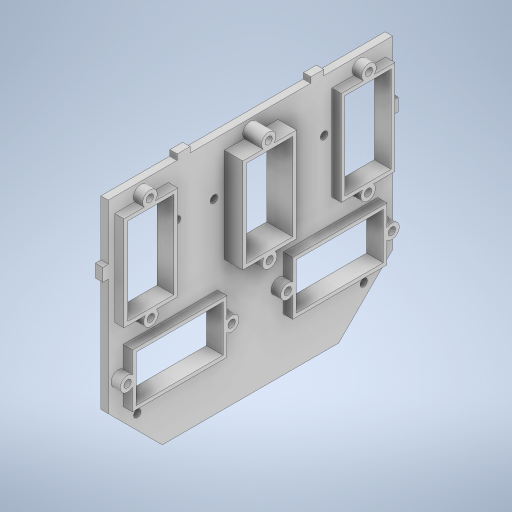
# Autodesk Inventor part: Palm_ServoAttachment
Saved by Autodesk Inventor 2023 (Build 270158000, 158)
## iProperties
Created: 2023-04-20
Part Number: Palm_ServoAttachment
Material: Generic
Document SubType Name: Modeling
Designer: 1senadi
Density: 1 g/cm^3
Appearance: Default
Author: 1senadi
Autodesk Inventor part; units mm, degrees
ref_plane "YZ Plane" through (0, 0, 0) normal (1, 0, 0) x (0, 1, 0)
ref_plane "XZ Plane" through (0, 0, 0) normal (0, 1, 0) x (-1, 0, 0)
ref_plane "XY Plane" through (0, 0, 0) normal (0, 0, 1) x (1, 0, 0)
sketch "Sketch1" plane through (0, 0, 0) normal (1, 0, 0) x (0, 1, 0)
  line L0 (0, 0) -> (0, -76.8)
  line L1 (0, 0) -> (76.8, 0) construction
  line L2 (0, -76.8) -> (-50, -76.8)
  line L3 (-50, -76.8) -> (-50, 0)
  line L4 (-50, 0) -> (0, 0)
  dimension "d0" = 76.8
  dimension "d1" = 90
  dimension "d2" = 50
  constraints: 10 end point, 3 perpendicular, 2 horizontal, 1 vertical
  measures "d0" distance of L0.start L0.end
  measures "d1" angle of L0 L1
  measures "d2" distance of L0.end L2.end
extrude "Extrusion1" add sketch "Sketch1" along normal blind 2
sketch "Sketch2" plane through (0, 0, 0) normal (-1, 0, 0) x (0, 0, 1)
  line L0 (-76.8, -50) -> (-76.8, 0) projected
  line L1 (-76.8, 0) -> (-73.92, 0)
  line L2 (-76.8, 0) -> (0, 0) projected
  line L3 (-73.92, 0) -> (-73.92, -5)
  line L4 (-73.92, -5) -> (-61.42, -5)
  line L5 (-61.42, -5) -> (-61.42, -28.5)
  line L6 (-61.42, -28.5) -> (-73.92, -28.5)
  line L7 (-73.92, -28.5) -> (-73.92, -5)
  line L8 (-73.92, -5) -> (-38.32, -5)
  line L9 (-38.32, -5) -> (-2.72, -5)
  line L10 (-2.72, -5) -> (-2.72, -28.5)
  line L11 (-2.72, -28.5) -> (-15.22, -28.5)
  line L12 (-15.22, -28.5) -> (-15.22, -5)
  line L13 (-38.32, -5) -> (-32.32, -5)
  line L14 (-32.32, -5) -> (-32.32, -28.5)
  line L15 (-32.32, -28.5) -> (-44.82, -28.5)
  line L16 (-44.82, -28.5) -> (-44.82, -5)
  line L17 (-67.67, -28.5) -> (-67.67, -30.813)
  line L18 (-67.92, -5) -> (-67.92, -2.687)
  circle A0 centre (-67.92, -2.687) radius 1
  circle A1 centre (-67.67, -30.813) radius 1
  line L19 (-38.57, -28.5) -> (-38.57, -30.813)
  line L20 (-38.32, -5) -> (-38.32, -2.687)
  line L21 (-8.72, -5) -> (-8.72, -2.687)
  line L22 (-8.97, -28.5) -> (-8.97, -30.813)
  circle A2 centre (-38.32, -2.687) radius 1
  circle A3 centre (-8.72, -2.687) radius 1
  circle A4 centre (-38.57, -30.813) radius 1
  circle A5 centre (-8.97, -30.813) radius 1
  dimension "d5" = 2.88
  dimension "d6" = 5
  dimension "d7" = 12.5
  dimension "d8" = 23.5
  dimension "d9" = 12.5
  dimension "d10" = 35.6
  dimension "d14" = 35.6
  dimension "d15" = 23.5
  dimension "d16" = 12.5
  dimension "d17" = 6
  dimension "d18" = 23.5
  dimension "d19" = 12.5
  dimension "d24" = 2.313
  dimension "d25" = 2.313
  dimension "d26" = 2
  dimension "d27" = 2
  dimension "d28" = 2
  dimension "d29" = 2
  dimension "d30" = 2
  dimension "d31" = 2
  constraints: 42 end point, 9 perpendicular, 6 centre point, 6 coincident, 6 point on line, 6 vertical, 3 horizontal, 3 midpoint
  measures "d5" distance of L0.end L1.end
  measures "d6" distance of L1.end L3.end
  measures "d7" distance of L3.end L4.end
  measures "d8" distance of L4.end L5.end
  measures "d9" distance of L5.end L6.end
  measures "d10" distance of L3.end L8.end
  measures "d14" distance of L8.end L9.end
  measures "d15" distance of L9.end L10.end
  measures "d16" distance of L10.end L11.end
  measures "d17" distance of L8.end L13.end
  measures "d18" distance of L13.end L14.end
  measures "d19" distance of L14.end L15.end
  measures "d24" distance of L17.start L17.end
  measures "d25" distance of L18.start L18.end
  measures "d26" diameter of A0
  measures "d27" diameter of A1
  measures "d28" diameter of A2
  measures "d29" diameter of A3
  measures "d30" diameter of A4
  measures "d31" diameter of A5
extrude "Extrusion2" cut sketch "Sketch2" against normal up to surface (2 mm away)
sketch "Sketch8" plane through (2, 0, 0) normal (1, 0, 0) x (0, 0, -1)
  line L0 (0, 0) -> (0, -50) projected
  line L1 (0, 0) -> (0, -15)
  line L2 (0, -15) -> (0, -18.5)
  line L3 (0, -18.5) -> (-1.5, -18.5)
  line L4 (-1.5, -18.5) -> (-1.5, -15)
  line L5 (-1.5, -15) -> (0, -15)
  line L6 (0, 0) -> (18.6, 0)
  line L7 (76.8, 0) -> (0, 0) projected
  line L8 (18.6, 0) -> (22.1, 0)
  line L9 (22.1, 0) -> (22.1, 1.5)
  line L10 (22.1, 1.5) -> (18.6, 1.5)
  line L11 (18.6, 1.5) -> (18.6, 0)
  line L12 (0, -50) -> (76.8, -50) projected
  line L13 (38.4, -50) -> (38.4, 0)
  line L14 (76.8, -15) -> (76.8, -18.5)
  line L15 (76.8, -18.5) -> (78.3, -18.5)
  line L16 (78.3, -18.5) -> (78.3, -15)
  line L17 (78.3, -15) -> (76.8, -15)
  line L18 (58.2, 0) -> (54.7, 0)
  line L19 (54.7, 0) -> (54.7, 1.5)
  line L20 (54.7, 1.5) -> (58.2, 1.5)
  line L21 (58.2, 1.5) -> (58.2, 0)
  dimension "d63" = 15
  dimension "d64" = 3.5
  dimension "d65" = 1.5
  dimension "d66" = 3.5
  dimension "d67" = 18.6
  dimension "d68" = 3.5
  dimension "d69" = 1.5
  dimension "d70" = 3.5
  constraints: 38 end point, 8 symmetric about line, 5 point on line, 4 perpendicular, 1 midpoint, 1 parallel
  measures "d63" distance of L0.start L1.end
  measures "d64" distance of L1.end L2.end
  measures "d65" distance of L2.end L3.end
  measures "d66" distance of L3.end L4.end
  measures "d67" distance of L0.start L6.end
  measures "d68" distance of L6.end L8.end
  measures "d69" distance of L8.end L9.end
  measures "d70" distance of L9.end L10.end
extrude "Extrusion7" add sketch "Sketch8" against normal up to surface (2 mm away) contours L0 L3 L4 L5 | L11 L10 L9 L7 | L7 L19 L20 L21 | L17 L16 L15 L14
sketch "Sketch10" plane through (2, 0, 0) normal (1, 0, 0) x (0, 0, -1)
  circle A0 centre (8.97, -30.813) radius 1 projected
  line L0 (0, -18.5) -> (0, -50) projected
  line L1 (8.72, -31.813) -> (0, -31.813)
  line L2 (0, -31.813) -> (0, -36.813)
  line L3 (0, -36.813) -> (5, -36.813)
  line L4 (5, -36.813) -> (5, -49.313)
  line L5 (5, -49.313) -> (28.5, -49.313)
  line L6 (5, -49.313) -> (28.5, -49.313) construction
  line L7 (28.5, -49.313) -> (28.5, -36.813)
  line L8 (28.5, -36.813) -> (5, -36.813)
  line L9 (5, -43.063) -> (2.687, -43.063)
  line L10 (28.5, -43.063) -> (30.813, -43.063)
  circle A1 centre (2.687, -43.063) radius 1
  circle A2 centre (30.813, -43.063) radius 1
  line L11 (54.7, 0) -> (22.1, 0) projected
  line L12 (38.4, 0) -> (38.4, -50)
  line L13 (71.8, -36.813) -> (71.8, -49.313)
  line L14 (71.8, -49.313) -> (48.3, -49.313)
  line L15 (48.3, -49.313) -> (48.3, -36.813)
  line L16 (48.3, -36.813) -> (71.8, -36.813)
  line L17 (71.8, -43.063) -> (74.113, -43.063)
  line L18 (48.3, -43.063) -> (45.987, -43.063)
  circle A3 centre (74.113, -43.063) radius 1
  circle A4 centre (45.987, -43.063) radius 1
  point P0 (0, 0)
  dimension "d82" = 5
  dimension "d83" = 5
  dimension "d84" = 12.5
  dimension "d85" = 23.5
  dimension "d86" = 0
  dimension "d87" = 12.5
  dimension "d88" = 2.313
  dimension "d89" = 2.313
  dimension "d90" = 2
  dimension "d91" = 2
  constraints: 34 end point, 10 symmetric about line, 4 centre point, 4 coincident, 4 horizontal, 3 midpoint, 3 perpendicular, 2 point on line, 2 vertical, 1 collinear, 2 other
  measures "d82" distance of L1.end L2.end
  measures "d83" distance of L2.end L3.end
  measures "d84" distance of L3.end L4.end
  measures "d85" distance of L4.end L5.end
  measures "d86" distance between parallel lines of L5 L6
  measures "d87" distance of L5.end L7.end
  measures "d88" distance of L9.start L9.end
  measures "d89" distance of L10.start L10.end
  measures "d90" diameter of A1
  measures "d91" diameter of A2
extrude "Extrusion8" cut sketch "Sketch10" against normal up to surface (2 mm away) contours L8 L7 L5 L4 | A1 | A2 | L13 L14 L15 L16 | A3 | A4
sketch "Sketch11" plane through (2, 0, 0) normal (1, 0, 0) x (0, 0, -1)
  line L0 (0, -50) -> (76.8, -50) projected
  line L1 (0, -50) -> (14.5664, -64.5664)
  line L2 (0, -50) -> (20.6, -50) construction
  line L3 (76.8, -50) -> (62.2336, -64.5664)
  line L4 (76.8, -50) -> (97.4, -50) construction
  line L5 (62.2336, -64.5664) -> (14.5664, -64.5664)
  point P0 (0, 0)
  dimension "d94" = 20.6
  dimension "d95" = 45
  dimension "d96" = 20.6
  dimension "d97" = 135
  constraints: 10 end point, 2 equal length, 2 horizontal
  measures "d94" distance of L0.start L1.end
  measures "d95" angle of L1 L2
  measures "d96" distance of L0.end L3.end
  measures "d97" angle of L3 L4
extrude "Extrusion9" add sketch "Sketch11" against normal up to surface (2 mm away)
sketch "Sketch12" plane through (2, 0, 0) normal (1, 0, 0) x (0, 0, -1)
  circle A0 centre (2.687, -43.063) radius 1 projected
  circle A1 centre (30.813, -43.063) radius 1 projected
  line L0 (5, -36.813) -> (28.5, -36.813) projected
  line L1 (5, -49.313) -> (5, -36.813) projected
  line L2 (28.5, -49.313) -> (5, -49.313) projected
  line L3 (28.5, -36.813) -> (28.5, -49.313) projected
  line L4 (29.5, -35.813) -> (4, -35.813)
  line L5 (4, -35.813) -> (4, -50.313)
  line L6 (4, -50.313) -> (29.5, -50.313)
  line L7 (29.5, -50.313) -> (29.5, -35.813)
  circle A2 centre (2.687, -43.063) radius 2
  circle A3 centre (30.813, -43.063) radius 2
  point P0 (0, 0)
  point P1 (4, -41.313)
  point P2 (4, -44.313)
  point P3 (29.5, -41.313)
  point P4 (29.5, -44.313)
  point P5 (4, -44.5717)
  point P6 (4, -41.5543)
  point P7 (29.5, -41.5543)
  point P8 (29.5, -44.5717)
  dimension "d102" = 1
  dimension "d110" = 1
  dimension "d111" = 1
  constraints: 8 end point, 4 point on line, 2 centre point, 3 other
  measures "d102" distance between parallel lines of L0 L4
  measures "d110" radial gap between concentric circles of A0 A2
  measures "d111" radial gap between concentric circles of A1 A3
extrude "Extrusion10" add sketch "Sketch12" along normal blind 2.5
sketch "Sketch13" plane through (2, 0, 0) normal (1, 0, 0) x (0, 0, -1)
  line L0 (48.3, -49.313) -> (48.3, -36.813) projected
  line L1 (48.3, -36.813) -> (71.8, -36.813) projected
  line L2 (71.8, -49.313) -> (48.3, -49.313) projected
  line L3 (71.8, -36.813) -> (71.8, -49.313) projected
  circle A0 centre (74.113, -43.063) radius 1 projected
  circle A1 centre (45.987, -43.063) radius 1 projected
  line L4 (47.3, -35.813) -> (47.3, -50.313)
  line L5 (47.3, -50.313) -> (72.8, -50.313)
  line L6 (72.8, -50.313) -> (72.8, -35.813)
  line L7 (72.8, -35.813) -> (47.3, -35.813)
  arc A2 (47.3, -41.5543) -> (47.3, -44.5717) centre (45.987, -43.063) ccw
  arc A3 (72.8, -44.5717) -> (72.8, -41.5543) centre (74.113, -43.063) ccw
  point P0 (0, 0)
  dimension "d105" = 1
  dimension "d106" = 1
  dimension "d107" = 1
  constraints: 8 end point, 4 point on circle, 4 point on line, 2 centre point, 3 other
  measures "d105" distance between parallel lines of L0 L4
  measures "d106" radial gap between concentric circles of A1 A2
  measures "d107" radial gap between concentric circles of A0 A3
extrude "Extrusion11" add sketch "Sketch13" along normal blind 2.5
sketch "Sketch14" plane through (2, 0, 0) normal (1, 0, 0) x (0, 0, -1)
  line L0 (2.72, -5) -> (15.22, -5) projected
  line L1 (2.72, -28.5) -> (2.72, -5) projected
  line L2 (15.22, -28.5) -> (2.72, -28.5) projected
  circle A0 centre (8.97, -30.813) radius 1 projected
  line L3 (15.22, -5) -> (15.22, -28.5) projected
  circle A1 centre (8.72, -2.687) radius 1 projected
  line L4 (16.22, -29.5) -> (1.72, -29.5)
  line L5 (1.72, -29.5) -> (1.72, -4)
  line L6 (1.72, -4) -> (16.22, -4)
  line L7 (16.22, -4) -> (16.22, -29.5)
  circle A2 centre (8.72, -2.687) radius 2
  circle A3 centre (8.97, -30.813) radius 2
  point P0 (0, 0)
  point P1 (10.2287, -4)
  point P2 (7.2113, -4)
  point P3 (7.4613, -29.5)
  point P4 (10.4787, -29.5)
  dimension "d112" = 1
  dimension "d113" = 1
  dimension "d114" = 1
  constraints: 8 end point, 2 centre point, 3 other
  measures "d112" distance between parallel lines of L3 L7
  measures "d113" radial gap between concentric circles of A1 A2
  measures "d114" radial gap between concentric circles of A0 A3
extrude "Extrusion12" add sketch "Sketch14" along normal blind 2.5
sketch "Sketch15" plane through (2, 0, 0) normal (1, 0, 0) x (0, 0, -1)
  line L0 (32.32, -5) -> (44.82, -5) projected
  line L1 (44.82, -5) -> (44.82, -28.5) projected
  line L2 (32.32, -28.5) -> (32.32, -5) projected
  line L3 (44.82, -28.5) -> (32.32, -28.5) projected
  circle A0 centre (38.57, -30.813) radius 1 projected
  circle A1 centre (38.32, -2.687) radius 1 projected
  line L4 (45.82, -29.5) -> (45.82, -4)
  line L5 (45.82, -4) -> (31.32, -4)
  line L6 (31.32, -4) -> (31.32, -29.5)
  line L7 (31.32, -29.5) -> (45.82, -29.5)
  circle A2 centre (38.32, -2.687) radius 2
  circle A3 centre (38.57, -30.813) radius 2
  point P0 (0, 0)
  point P1 (39.8287, -4)
  point P2 (36.8113, -4)
  point P3 (37.0613, -29.5)
  point P4 (40.0787, -29.5)
  dimension "d117" = 1
  dimension "d118" = 1
  dimension "d119" = 1
  constraints: 8 end point, 2 centre point, 3 other
  measures "d117" distance between parallel lines of L1 L4
  measures "d118" radial gap between concentric circles of A1 A2
  measures "d119" radial gap between concentric circles of A0 A3
extrude "Extrusion13" add sketch "Sketch15" along normal blind 5
sketch "Sketch16" plane through (2, 0, 0) normal (1, 0, 0) x (0, 0, -1)
  line L0 (61.42, -5) -> (73.92, -5) projected
  line L1 (73.92, -5) -> (73.92, -28.5) projected
  line L2 (61.42, -28.5) -> (61.42, -5) projected
  line L3 (73.92, -28.5) -> (61.42, -28.5) projected
  circle A0 centre (67.67, -30.813) radius 1 projected
  circle A1 centre (67.92, -2.687) radius 1 projected
  line L4 (74.92, -4) -> (60.42, -4)
  line L5 (60.42, -4) -> (60.42, -29.5)
  line L6 (60.42, -29.5) -> (74.92, -29.5)
  line L7 (74.92, -29.5) -> (74.92, -4)
  circle A2 centre (67.92, -2.687) radius 2
  circle A3 centre (67.67, -30.813) radius 2
  point P0 (0, 0)
  point P1 (66.1613, -29.5)
  point P2 (69.1787, -29.5)
  point P3 (69.4287, -4)
  point P4 (66.4113, -4)
  dimension "d122" = 1
  dimension "d123" = 1
  dimension "d124" = 1
  constraints: 8 end point, 2 centre point, 3 other
  measures "d122" distance between parallel lines of L0 L4
  measures "d123" radial gap between concentric circles of A1 A2
  measures "d124" radial gap between concentric circles of A0 A3
extrude "Extrusion14" add sketch "Sketch16" along normal blind 2.5
sketch "Sketch17" plane through (0, 0, 0) normal (-1, 0, 0) x (0, 0, 1)
  line L0 (-14.5664, -64.5664) -> (-7.7937, -57.7937)
  line L1 (-14.5664, -64.5664) -> (0, -50) projected
  line L2 (-7.7937, -57.7937) -> (-7.7937, -53.7937)
  circle A0 centre (-7.7937, -53.7937) radius 1
  line L3 (-14.5664, -64.5664) -> (-62.2336, -64.5664) projected
  line L4 (-38.4, -64.5664) -> (-38.4, 0)
  line L5 (-54.7, 0) -> (-22.1, 0) projected
  circle A1 centre (-69.0063, -53.7937) radius 1
  point P0 (0, 0)
  dimension "d127" = 9.578
  dimension "d128" = 4
  dimension "d129" = 2
  constraints: 6 end point, 2 centre point, 2 midpoint, 1 coincident, 1 point on line, 1 symmetric about line, 1 vertical, 1 other
  measures "d127" distance of L0.start L0.end
  measures "d128" distance of L0.end L2.end
  measures "d129" diameter of A0
extrude "Extrusion15" cut sketch "Sketch17" against normal up to surface (2 mm away)
sketch "Sketch18" plane through (0, 0, 0) normal (-1, 0, 0) x (0, 0, 1)
  line L0 (-18.6, 0) -> (0, 0) projected
  line L1 (0, 0) -> (-23.52, 0)
  line L2 (-23.52, 0) -> (-23.52, -14)
  line L3 (-62.2336, -64.5664) -> (-14.5664, -64.5664) projected
  line L4 (-38.4, -64.5664) -> (-38.4, 0)
  line L5 (-54.7, 0) -> (-22.1, 0) projected
  line L6 (0, 0) -> (-38.4, 0)
  line L7 (-23.52, -14) -> (-18.52, -14)
  line L8 (-23.52, -14) -> (-28.52, -14)
  circle A0 centre (-18.52, -14) radius 1
  circle A1 centre (-28.52, -14) radius 1
  circle A2 centre (-58.28, -14) radius 1
  dimension "d132" = 23.52
  dimension "d133" = 14
  dimension "d135" = 38.4
  dimension "d136" = 5
  dimension "d137" = 5
  dimension "d138" = 2
  dimension "d139" = 2
  constraints: 12 end point, 3 centre point, 3 horizontal, 2 coincident, 2 midpoint, 1 point on line, 1 symmetric about line, 1 vertical, 1 other
  measures "d132" distance of L0.end L1.end
  measures "d133" distance of L1.end L2.end
  measures "d135" distance of L0.end L4.end
  measures "d136" distance of L2.end L7.end
  measures "d137" distance of L2.end L8.end
  measures "d138" diameter of A0
  measures "d139" diameter of A1
extrude "Extrusion16" cut sketch "Sketch18" against normal up to surface (2 mm away)
body "Solid1"
